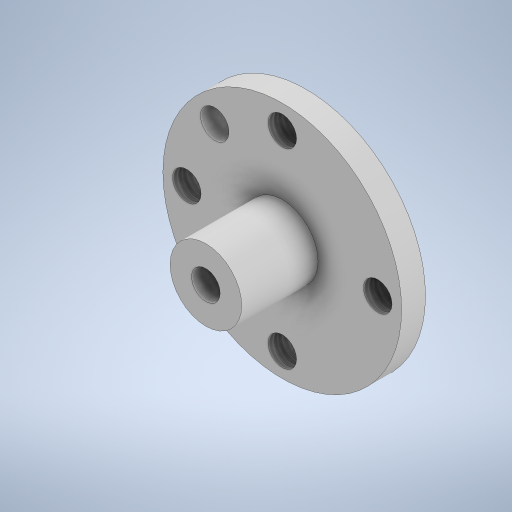
# Autodesk Inventor part: Base
Saved by Autodesk Inventor 2023 (Build 270158000, 158)
## iProperties
Created: 2022-08-22
Part Number: Base
Material: Generic
Document SubType Name: Modeling
Designer: ivanm
Density: 1 g/cm^3
Appearance: Default
Author: ivanm
Autodesk Inventor part; units mm, degrees
ref_plane "YZ Plane" through (0, 0, 0) normal (1, 0, 0) x (0, 1, 0)
ref_plane "XZ Plane" through (0, 0, 0) normal (0, 1, 0) x (-1, 0, 0)
ref_plane "XY Plane" through (0, 0, 0) normal (0, 0, 1) x (1, 0, 0)
sketch "Sketch1" plane through (0, 0, 0) normal (0, 0, 1) x (1, 0, 0)
  circle A0 centre (0, 0) radius 25
  dimension "d0" = 50
  constraints: 1 centre point, 1 coincident
  measures "d0" diameter of A0
extrude "Extrusion1" add sketch "Sketch1" along normal blind 5
sketch "Sketch2" plane through (0, 0, 5) normal (0, 0, 1) x (1, 0, 0)
  circle A0 centre (0, 20) radius 3
  circle A1 centre (20, 0) radius 3
  circle A2 centre (-20, 0) radius 3
  circle A3 centre (0, -20) radius 3
  dimension "d4" = 6
  dimension "d5" = 6
  dimension "d6" = 6
  dimension "d7" = 6
  constraints: 4 centre point
  measures "d4" diameter of A0
  measures "d5" diameter of A1
  measures "d6" diameter of A2
  measures "d7" diameter of A3
hole "Hole1" at (-20, 0, 5) at (0, 20, 5) at (20, 0, 5) at (0, -20, 5) direction (0, 0, -1) diameter 6 end through all
thread "Thread1" size "M6x1" class "6H" standard "ANSI Metric M Profile" full length
thread "Thread2" size "M6x1" class "6H" standard "ANSI Metric M Profile" full length
thread "Thread3" size "M6x1" class "6H" standard "ANSI Metric M Profile" full length
thread "Thread4" size "M6x1" class "6H" standard "ANSI Metric M Profile" full length
pattern_circular "Circular Pattern1" count 2 over 45 about axis through (0, 0, 0) along (0, 0, 1) of "Hole1"
sketch "Sketch4" plane through (0, 0, 5) normal (0, 0, 1) x (1, 0, 0)
  circle A0 centre (14.1421, 14.1421) radius 3 projected
  circle A1 centre (14.1421, 14.1421) radius 3
  circle A2 centre (14.1421, -14.1421) radius 3 projected
  circle A3 centre (14.1421, -14.1421) radius 3
  circle A4 centre (-14.1421, -14.1421) radius 3 projected
  circle A5 centre (-14.1421, -14.1421) radius 3
  point P0 (0, 0)
  constraints: 3 centre point, 3 coincident
extrude "Extrusion2" add sketch "Sketch4" against normal blind 5
sketch "Sketch5" plane through (0, 0, 5) normal (0, 0, 1) x (1, 0, 0)
  circle A0 centre (-14.1421, 14.1421) radius 3 projected
  circle A1 centre (20, 0) radius 3 projected
  circle A2 centre (-20, 0) radius 3 projected
  circle A3 centre (0, 20) radius 3 projected
  circle A4 centre (0, -20) radius 3 projected
  circle A5 centre (0, 0) radius 25 projected
  circle A6 centre (0, 0) radius 7.5
  circle A7 centre (0, 0) radius 3
  dimension "d29" = 15
  dimension "d30" = 6
  constraints: 2 centre point, 2 coincident
  measures "d29" diameter of A6
  measures "d30" diameter of A7
extrude "Extrusion3" add sketch "Sketch5" along normal blind 16 contours A6
body "Solid1"
